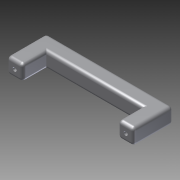
# Autodesk Inventor part: maneta porta
Saved by Autodesk Inventor 2012 SP1 (Build 160190100, 190)
## iProperties
Created: 2015-03-29
Part Number: maneta porta
Material: Default
Document SubType Name: Modeling
Designer: sheina
Density: 1 g/cm^3
Author: sheina
Autodesk Inventor part; units mm, degrees
ref_plane "YZ Plane" through (0, 0, 0) normal (1, 0, 0) x (0, 1, 0)
ref_plane "XZ Plane" through (0, 0, 0) normal (0, 1, 0) x (-1, 0, 0)
ref_plane "XY Plane" through (0, 0, 0) normal (0, 0, 1) x (1, 0, 0)
sketch "Boceto1" plane through (0, 0, 0) normal (0, 0, 1) x (1, 0, 0)
  line L0 (0, 0) -> (80, 0)
  line L1 (80, 0) -> (80, -25)
  line L2 (80, -25) -> (70, -25)
  line L3 (70, -25) -> (70, -10)
  line L4 (70, -10) -> (10, -10)
  line L5 (10, -10) -> (10, -25)
  line L6 (10, -25) -> (0, -25)
  line L7 (0, -25) -> (0, 0)
  dimension "d0" = 10
  dimension "d1" = 80
  dimension "d2" = 10
  dimension "d3" = 15
  dimension "d4" = 25
  dimension "d6" = 25
  constraints: 16 end point, 6 parallel, 1 horizontal, 1 perpendicular
  measures "d0" distance between parallel lines of L5 L7
  measures "d1" distance between parallel lines of L7 L1
  measures "d2" distance between parallel lines of L1 L3
  measures "d3" distance from line of L4 L5.end
  measures "d4" distance from line of L0 L1.end
  measures "d6" distance from line of L0 L5.end
extrude "Extrusión1" add sketch "Boceto1" along normal blind 10
fillet "Empalme1" radius 2 21 edges at (10, -17.5, 10) (40, -10, 10) (70, -17.5, 10) (10, -17.5, 0) (40, -10, 0) (70, -25, 5) (75, -25, 10) (75, -25, 0) (80, -25, 5) (80, -12.5, 10) (80, -12.5, 0) (40, 0, 10) (0, -12.5, 10) (5, -25, 10) (0, -25, 5) (5, -25, 0) (40, 0, 0) (80, 0, 5) (0, 0, 5) (0, -12.5, 0) (70, -17.5, 0)
sketch "Boceto2" plane through (72, -25, 8) normal (0, -1, 0) x (1, 0, 0)
  circle A0 centre (3, -3) radius 1.25
  point P0 (-72, -8)
  dimension "d10" = 2.5
  constraints: 1 centre point
  measures "d10" diameter of A0
extrude "Extrusión2" cut sketch "Boceto2" against normal blind 12
fillet "Empalme2" radius 2 3 edges at (9.4142, -24.4142, 9.4142) (9.4142, -24.4142, 0.5858) (10, -25, 5)
sketch "Boceto4" plane through (2, -25, 2) normal (0, -1, 0) x (1, 0, 0)
  circle A0 centre (3, 3) radius 1.25
  point P0 (-2, -2)
  dimension "d18" = 2.5
  constraints: 1 centre point
  measures "d18" diameter of A0
extrude "Extrusión4" cut sketch "Boceto4" against normal blind 12
